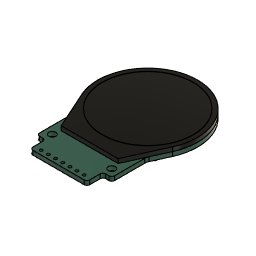
LCD Round 1.3_ SPI v1 (Autodesk Fusion 360 design; units mm, degrees)
Autodesk Fusion 360 part; units mm, degrees
note: some values were not read from the file. Set by a fixed rule: which sketch regions a step uses.
sketch "PCB Board" plane through (0, 0, 0) normal (0, 0, 1) x (1, 0, 0) in component "PCB"
  circle A0 centre (0, 0) radius 17.75 construction
  line L0 (-13.3, -31.8) -> (13.3, -31.8) construction
  line L1 (13.3, -31.8) -> (13.3, 0) construction
  line L2 (13.3, 0) -> (-13.3, 0) construction
  line L3 (-13.3, 0) -> (-13.3, -31.8) construction
  circle A1 centre (-10.6, -23.4) radius 1.25
  line L4 (0, 20) -> (0, -35)
  circle A2 centre (10.6, -23.4) radius 1.25
  circle A3 centre (-10.6, -23.4) radius 2.7 construction
  circle A4 centre (10.6, -23.4) radius 2.7 construction
  line L5 (-10.14, -31.8) -> (10.14, -31.8) construction
  line L6 (10.14, -31.8) -> (10.14, -26.1) construction
  line L7 (10.14, -26.1) -> (-10.14, -26.1) construction
  line L8 (-10.14, -26.1) -> (-10.14, -31.8) construction
  line L9 (-10.14, -26.1) -> (10, -26.1) construction
  line L10 (10, -26.1) -> (10, -20.7) construction
  line L11 (10, -20.7) -> (-10.14, -20.7) construction
  line L12 (-10.14, -20.7) -> (-10.14, -26.1) construction
  line L13 (-10.14, -20.7) -> (-16.1824, -7.2934) construction
  line L14 (10.14, -20.7) -> (16.1824, -7.2934) construction
  line L15 (-16.2663, -7.1072) -> (-13.3, -13.6887)
  line L16 (-13.3, -13.6887) -> (-13.3, -26.2843)
  line L17 (-13.3, -26.2843) -> (-10.14, -26.2843)
  line L18 (-10.14, -26.2843) -> (-10.14, -31.8)
  line L19 (-10.14, -31.8) -> (10.14, -31.8)
  line L20 (10.14, -31.8) -> (10.14, -26.1)
  line L21 (10.14, -26.1) -> (13.3, -26.1)
  line L22 (13.3, -26.1) -> (13.3, -13.6887)
  line L23 (13.3, -13.6887) -> (16.1824, -7.2934)
  arc A5 (16.1824, -7.2934) -> (-16.2663, -7.1072) centre (-0.0006, 0.0003) ccw
  line L24 (-7.64, -32.5) -> (-7.64, -27.5) construction
  line L25 (-10.5, -30.3) -> (10.5, -30.3) construction
  circle A6 centre (-7.64, -30.3) radius 0.5
  circle A7 centre (-5.0933, -30.3) radius 0.5
  circle A8 centre (-2.5467, -30.3) radius 0.5
  circle A9 centre (0, -30.3) radius 0.5
  circle A10 centre (2.5467, -30.3) radius 0.5
  circle A11 centre (5.0933, -30.3) radius 0.5
  circle A12 centre (7.64, -30.3) radius 0.5
  dimension "d1" = 35.5
  dimension "d2" = 26.6
  dimension "d3" = 31.8
  dimension "d5" = 2.5
  dimension "d6" = 8.4
  dimension "d7" = 21.2
  dimension "d8" = 20.28
  dimension "d18" = 2.5
  dimension "d19" = 1.5
  dimension "d20" = 1
  dimension "d23" = 15.28
  dimension "d24" = 0
  constraint coincident A0.centre origin
  constraint horizontal L0
  constraint vertical L1
  constraint horizontal L2
  constraint vertical L3
  constraint midpoint A0.centre L2
  constraint perpendicular L0 L4
  constraint symmetric A1 L4 A2
  constraint concentric A1 A3
  constraint tangent L3 A3
  constraint concentric A2 A4
  constraint tangent L1 A4
  constraint horizontal L5
  constraint vertical L6
  constraint horizontal L7
  constraint vertical L8
  constraint midpoint L0 L5
  constraint tangent A3 L7
  constraint horizontal L9
  constraint vertical L10
  constraint horizontal L11
  constraint vertical L12
  constraint tangent A3 L11
  constraint coincident A0 L13.end
  constraint tangent A0 L13
  constraint symmetric L4 L11.end L14.start
  constraint symmetric L4 L13.end L14.end
  constraint coincident L13 L15.end
  constraint coincident L3 L15.end
  constraint parallel L13 L15
  constraint coincident L3 L16.end
  constraint coincident L8 L17.end
  constraint perpendicular L8 L17
  constraint perpendicular L0 L18
  constraint coincident L1 L21.end
  constraint perpendicular L1 L21
  constraint coincident L14 L22.end
  constraint coincident L1 L22.end
  constraint tangent A0 L23
  constraint tangent A0 A5
  constraint perpendicular L0 L24
  constraint perpendicular L20 L25
  constraint coincident L25 A6.centre
  constraint coincident L24 A6.centre
  measures "d1" diameter of A0
  measures "d2" distance of L0.start L0.end
  measures "d3" distance of L0.start L2.end
  measures "d5" diameter of A1
  measures "d6" distance of L0 A1.centre
  measures "d7" distance of A1.centre A2.centre
  measures "d8" distance of L5.start L5.end
  measures "d18" distance of L18 L24
  measures "d19" distance of L5 L25
  measures "d20" diameter of A6
extrude "Extrude1" add sketch "PCB Board" along normal blind 1.5 contours L4 L19 L20 L21 L22 L23 A5 A9 | L4 L15 L16 L17 L18 L19 A5 A9 makes body 1 in component "PCB"
sketch "Components" plane through (0, 0, 0) normal (0, 0, -1) x (1, 0, 0) in component "PCB"
  circle A0 centre (-10.6, 23.4) radius 1.25
  circle A1 centre (10.6, 23.4) radius 1.25
  arc A2 (-16.2663, 7.1072) -> (16.1824, 7.2934) centre (-0.0006, -0.0003) ccw
  line L0 (16.1824, 7.2934) -> (13.3, 13.6887)
  line L1 (13.3, 13.6887) -> (13.3, 26.1)
  line L2 (13.3, 26.1) -> (10.14, 26.1)
  line L3 (10.14, 26.1) -> (10.14, 31.8)
  line L4 (10.14, 31.8) -> (-10.14, 31.8)
  line L5 (-10.14, 31.8) -> (-10.14, 26.2843)
  line L6 (-10.14, 26.2843) -> (-13.3, 26.2843)
  line L7 (-13.3, 26.2843) -> (-13.3, 13.6887)
  line L8 (-13.3, 13.6887) -> (-16.2663, 7.1072)
  line L9 (-12.5055, 9.8) -> (12.4945, 9.8)
  line L10 (12.4945, 9.8) -> (12.4945, -3.2)
  line L11 (12.4945, -3.2) -> (-12.5055, -3.2)
  line L12 (-12.5055, -3.2) -> (-12.5055, 9.8)
  line L13 (-0.0055, -22.0727) -> (-0.0055, 33.9952)
  circle A3 centre (7.64, 30.3) radius 0.5
  circle A4 centre (2.5467, 30.3) radius 0.5
  circle A5 centre (-2.5467, 30.3) radius 0.5
  circle A6 centre (0, 30.3) radius 0.5
  circle A7 centre (-5.0933, 30.3) radius 0.5
  circle A8 centre (5.0933, 30.3) radius 0.5
  circle A9 centre (-7.64, 30.3) radius 0.5
  dimension "d12" = 13
  dimension "d13" = 22
  dimension "d15" = 25
  constraint horizontal L9
  constraint vertical L10
  constraint horizontal L11
  constraint vertical L12
  measures "d12" distance of L9.start L11.end
  measures "d13" distance of L4 L9
  measures "d15" distance of L10.end L11.end
extrude "Extrude2" add sketch "Components" along normal blind 2 contours L9 L10 L11 L13 | L9 L11 L12 L13 bodies 1 in component "PCB"
sketch "Display" plane through (0, 0, 1.5) normal (0, 0, 1) x (1, 0, 0) in component "Display"
  line L0 (-10.14, -20.7) -> (-16.1824, -7.2934)
  line L1 (10, -20.7) -> (-10.14, -20.7)
  line L2 (10.14, -20.7) -> (16.1824, -7.2934)
  arc A0 (16.1824, -7.2934) -> (-16.2663, -7.1072) centre (-0.0006, 0.0003) ccw
  arc A1 (16.1824, -7.2934) -> (-16.1824, -7.2934) centre (0, 0.0007) ccw
  line L3 (-16.2663, -7.1072) -> (-10.14, -20.7)
  line L4 (-10.14, -20.7) -> (10.14, -20.7)
  line L5 (10.14, -20.7) -> (16.1824, -7.2934)
  circle A2 centre (7.64, -30.3) radius 0.5
  circle A3 centre (2.5467, -30.3) radius 0.5
  circle A4 centre (-2.5467, -30.3) radius 0.5
  circle A5 centre (0, -30.3) radius 0.5
  circle A6 centre (10.6, -23.4) radius 1.25
  circle A7 centre (-5.0933, -30.3) radius 0.5
  circle A8 centre (-10.6, -23.4) radius 1.25
  circle A9 centre (5.0933, -30.3) radius 0.5
  circle A10 centre (-7.64, -30.3) radius 0.5
  arc A11 (16.1824, -7.2934) -> (-16.2663, -7.1072) centre (-0.0006, 0.0003) ccw
  line L6 (-16.2663, -7.1072) -> (-13.3, -13.6887)
  line L7 (-13.3, -13.6887) -> (-13.3, -26.2843)
  line L8 (-13.3, -26.2843) -> (-10.14, -26.2843)
  line L9 (-10.14, -26.2843) -> (-10.14, -31.8)
  line L10 (-10.14, -31.8) -> (10.14, -31.8)
  line L11 (10.14, -31.8) -> (10.14, -26.1)
  line L12 (10.14, -26.1) -> (13.3, -26.1)
  line L13 (13.3, -26.1) -> (13.3, -13.6887)
  line L14 (13.3, -13.6887) -> (16.1824, -7.2934)
  constraint coincident L2.end A0.start
  constraint coincident L0.end A1.end
  constraint coincident A0.end L3.start
  constraint coincident L0.start L1.end
  constraint coincident L2.start L4.end
extrude "Extrude1'" add sketch "Display" along normal blind 1.5 separate body contours L0 L1 L2 A0 A1 L3 L4 L5 A11 L6 L14 makes body 2 in component "Display"
sketch "Visible" plane through (0, 0, 3) normal (0, 0, 1) x (-1, 0, 0) in component "Display"
  line L0 (-10.14, 20.7) -> (-16.1824, 7.2934)
  arc A0 (-16.1824, 7.2934) -> (16.1824, 7.2934) centre (0, -0.0007) ccw
  line L1 (16.1824, 7.2934) -> (10.14, 20.7)
  line L2 (10.14, 20.7) -> (-10.14, 20.7)
  circle A1 centre (0, 0) radius 16.2
  dimension "d27" = 32.4
  constraint coincident A1.centre origin
  measures "d27" diameter of A1
extrude "Extrude2'" add sketch "Visible" along normal blind 0.1 contours A1 bodies 2 in component "Display"
fillet "Fillet1" radius 1 6 edges at (10.14, -31.8, 0.75) (-10.14, -31.8, 0.75) (10.14, -26.1, 0.75) (13.3, -26.1, 0.75) (-10.14, -26.2843, 0.75) (-13.3, -26.2843, 0.75) on bodies 1 in component "PCB"
fillet "Fillet2" radius 3 2 edges at (-13.3, -13.6887, 0.75) (13.3, -13.6887, 0.75) on bodies 1 in component "PCB"
component "PCB" placed x (1, 0, 0) y (0, 1, 0) z (0, 0, 1) at (0, 0, 0)
component "Display" placed x (1, 0, 0) y (0, 1, 0) z (0, 0, 1) at (0, 0, 0)
